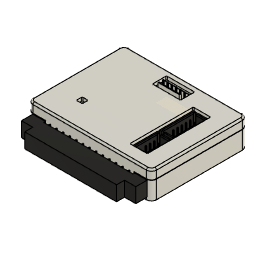
VIC20_Diag_UP_PCB_v0 v8 (Autodesk Fusion 360 design; units mm, degrees)
Autodesk Fusion 360 part; units mm, degrees
(part 1 of 2)
sketch "DXF import" plane through (0, 0, 0) normal (0, 0, 1) x (1, 0, 0) in component "PCB"
  arc A0 (0, 1) -> (1, 0) centre (1, 1) ccw
  line L0 (53, 1) -> (53, 54)
  line L1 (0, 1) -> (0, 54)
  arc A1 (53, 54) -> (52, 55) centre (52, 54) ccw
  line L2 (52, 55) -> (1, 55)
  line L3 (1, 0) -> (52, 0)
  arc A2 (1, 55) -> (0, 54) centre (1, 54) ccw
  arc A3 (52, 0) -> (53, 1) centre (52, 1) ccw
  circle A4 centre (4, 51) radius 3.1
  line L4 (50.18, 0) -> (50.18, -1)
  circle A5 centre (49, 51) radius 3.1
  line L5 (46.72, -1) -> (46.72, 0)
  circle A6 centre (49, 51) radius 1.5875
  line L6 (46.72, 0) -> (46.22, 0)
  line L7 (49.45, 0.1) -> (49.45, -1)
  line L8 (47.45, 0.1) -> (47.45, -1)
  line L9 (46.22, 0) -> (46.22, -1)
  line L10 (50.68, -1) -> (50.68, 0)
  line L11 (50.68, 0) -> (50.18, 0)
  line L12 (31.61, 0.1) -> (31.61, -1)
  circle A7 centre (4, 51) radius 1.5875
  line L13 (22.96, 0) -> (22.46, 0)
  line L14 (7.85, 0.1) -> (7.85, -1)
  line L15 (42.76, -1) -> (42.76, 0)
  line L16 (43.49, 0.1) -> (43.49, -1)
  line L17 (45.49, 0.1) -> (45.49, -1)
  line L18 (30.88, -1) -> (30.88, 0)
  line L19 (7.12, -1) -> (7.12, 0)
  line L20 (22.46, 0) -> (22.46, -1)
  line L21 (7.12, 0) -> (6.62, 0)
  line L22 (35.57, 0.1) -> (35.57, -1)
  line L23 (6.62, 0) -> (6.62, -1)
  line L24 (14.54, 0) -> (14.54, -1)
  line L25 (37.57, 0.1) -> (37.57, -1)
  line L26 (38.8, -1) -> (38.8, 0)
  line L27 (15.04, 0) -> (14.54, 0)
  line L28 (18.5, 0) -> (18.5, -1)
  line L29 (29.65, 0.1) -> (29.65, -1)
  line L30 (30.88, 0) -> (30.38, 0)
  line L31 (27.65, 0.1) -> (27.65, -1)
  line L32 (26.42, 0) -> (26.42, -1)
  line L33 (38.8, 0) -> (38.3, 0)
  line L34 (34.84, 0) -> (34.34, 0)
  line L35 (39.53, 0.1) -> (39.53, -1)
  line L36 (42.26, 0) -> (42.26, -1)
  line L37 (42.76, 0) -> (42.26, 0)
  line L38 (26.92, -1) -> (26.92, 0)
  line L39 (38.3, 0) -> (38.3, -1)
  line L40 (33.61, 0.1) -> (33.61, -1)
  line L41 (34.34, 0) -> (34.34, -1)
  line L42 (26.92, 0) -> (26.42, 0)
  line L43 (30.38, 0) -> (30.38, -1)
  line L44 (34.84, -1) -> (34.84, 0)
  line L45 (41.53, 0.1) -> (41.53, -1)
  line L46 (21.73, 0.1) -> (21.73, -1)
  line L47 (15.77, 0.1) -> (15.77, -1)
  line L48 (11.08, -1) -> (11.08, 0)
  line L49 (23.69, 0.1) -> (23.69, -1)
  line L50 (19.73, 0.1) -> (19.73, -1)
  line L51 (25.69, 0.1) -> (25.69, -1)
  line L52 (19, -1) -> (19, 0)
  line L53 (11.81, 0.1) -> (11.81, -1)
  line L54 (54.17, -6.8) -> (54.17, -11.6)
  line L55 (11.08, 0) -> (10.58, 0)
  line L56 (22.96, -1) -> (22.96, 0)
  line L57 (55.97, -6.8) -> (54.17, -6.8)
  line L58 (-6.03, -6.8) -> (-7.58, -6.8)
  line L59 (59.37, -6.8) -> (55.97, -6.8)
  line L60 (60.92, -6.8) -> (59.37, -6.8)
  line L61 (19, 0) -> (18.5, 0)
  line L62 (9.85, 0.1) -> (9.85, -1)
  line L63 (53.47, 0) -> (53.47, -1)
  line L64 (3.16, -1) -> (3.16, 0)
  line L65 (17.77, 0.1) -> (17.77, -1)
  line L66 (-2.63, -6.8) -> (-2.63, -5.2)
  line L67 (-4.33, 0) -> (-4.33, -2.8667)
  line L68 (57.67, -3.6853) -> (57.67, -3.548)
  line L69 (55.97, -4.2) -> (55.97, -2.6)
  line L70 (59.37, -1.6) -> (59.37, 0)
  line L71 (60.92, 0) -> (59.37, 0)
  line L72 (59.37, 0) -> (57.67, 0)
  line L73 (-4.33, -3.548) -> (-4.33, -3.6853)
  line L74 (-4.33, -4.3667) -> (-4.33, -7.2333)
  line L75 (55.97, -1.6) -> (55.97, 0)
  line L76 (57.67, 0) -> (55.97, 0)
  line L77 (-0.83, -6.8) -> (-2.63, -6.8)
  line L78 (-2.63, -4.2) -> (-2.63, -2.6)
  line L79 (-4.33, -8.7333) -> (-4.33, -11.6)
  line L80 (-4.33, 0) -> (-6.03, 0)
  line L81 (10.58, 0) -> (10.58, -1)
  line L82 (13.81, 0.1) -> (13.81, -1)
  line L83 (5.89, 0.1) -> (5.89, -1)
  line L84 (-2.63, -1.6) -> (-2.63, 0)
  line L85 (-6.03, -1.6) -> (-6.03, 0)
  line L86 (55.97, 0) -> (53.47, 0)
  line L87 (-7.58, 0) -> (-7.58, -6.8)
  line L88 (3.16, 0) -> (2.66, 0)
  line L89 (3.89, 0.1) -> (3.89, -1)
  line L90 (15.04, -1) -> (15.04, 0)
  line L91 (59.37, -4.2) -> (59.37, -2.6)
  line L92 (-6.03, -6.8) -> (-6.03, -5.2)
  line L93 (2.66, 0) -> (2.66, -1)
  line L94 (51.81, 14.73) -> (52.6038, 14.73)
  line L95 (52.6038, 23.62) -> (52.6038, 17.27)
  line L96 (-0.13, 0) -> (-2.63, 0)
  line L97 (60.92, 0) -> (60.92, -6.8)
  line L98 (46.2537, 8.38) -> (44.825, 8.38)
  line L99 (51.81, 17.27) -> (52.6038, 17.27)
  line L100 (-0.83, -11.6) -> (-0.83, -6.8)
  line L101 (-6.03, 0) -> (-7.58, 0)
  line L102 (57.67, -2.8667) -> (57.67, 0)
  line L103 (51.3338, 17.27) -> (51.81, 17.27)
  line L104 (46.2537, 23.62) -> (52.6038, 23.62)
  line L105 (44.6662, 22.35) -> (44.825, 22.35)
  line L106 (51.3338, 9.65) -> (46.2537, 9.65)
  line L107 (44.825, 22.35) -> (44.825, 22.8263)
  line L108 (57.67, -11.6) -> (57.67, -8.7333)
  line L109 (43.3962, 23.62) -> (44.825, 23.62)
  line L110 (51.81, 14.73) -> (51.81, 9.1737)
  line L111 (46.2537, 22.35) -> (46.2537, 22.8263)
  line L112 (57.67, -7.2333) -> (57.67, -4.3667)
  line L113 (44.825, 8.38) -> (43.3962, 8.38)
  line L114 (51.3338, 22.35) -> (51.3338, 17.27)
  line L115 (44.825, 9.65) -> (44.825, 9.1737)
  line L116 (55.97, -6.8) -> (55.97, -5.2)
  line L117 (51.3338, 22.35) -> (51.81, 22.8263)
  line L118 (51.3338, 14.73) -> (51.3338, 9.65)
  line L119 (-4.33, -7.9147) -> (-4.33, -8.052)
  line L120 (53.47, -1) -> (-0.13, -1)
  line L121 (-2.63, -6.8) -> (-6.03, -6.8)
  line L122 (44.6662, 9.65) -> (44.6662, 22.35)
  line L123 (46.2537, 22.35) -> (51.3338, 22.35)
  line L124 (54.17, -11.6) -> (-0.83, -11.6)
  line L125 (57.67, -8.052) -> (57.67, -7.9147)
  line L126 (52.6038, 14.73) -> (52.6038, 8.38)
  line L127 (51.3338, 17.27) -> (51.3338, 14.73)
  line L128 (43.3962, 8.38) -> (43.3962, 23.62)
  line L129 (46.2537, 9.65) -> (44.825, 9.65)
  line L130 (51.3338, 14.73) -> (51.81, 14.73)
  line L131 (-6.03, -4.2) -> (-6.03, -2.6)
  line L132 (52.6038, 17.27) -> (52.6038, 14.73)
  line L133 (52.6038, 8.38) -> (46.2537, 8.38)
  line L134 (44.825, 9.65) -> (44.6662, 9.65)
  line L135 (59.37, -6.8) -> (59.37, -5.2)
  line L136 (44.825, 23.62) -> (46.2537, 23.62)
  line L137 (44.825, 22.35) -> (46.2537, 22.35)
  line L138 (-2.63, 0) -> (-4.33, 0)
  line L139 (-0.13, -1) -> (-0.13, 0)
  arc A8 (43.3962, 35.4763) -> (43.3962, 34.3651) centre (43.3962, 34.9207) ccw
  line L140 (46.2537, 9.1737) -> (51.81, 9.1737)
  line L141 (44.19, 9.1737) -> (44.6662, 9.65)
  arc A9 (43.3962, 10.92) -> (43.3962, 9.65) centre (43.3962, 10.285) ccw
  line L142 (44.825, 22.8263) -> (44.19, 22.8263)
  arc A10 (43.3962, 27.38) -> (43.3962, 26.11) centre (43.3962, 26.745) ccw
  line L143 (44.825, 24.84) -> (43.3962, 24.84)
  line L144 (44.825, 25.6337) -> (44.825, 24.84)
  line L145 (51.81, 25.6337) -> (51.3338, 26.11)
  arc A11 (43.3962, 22.35) -> (43.3962, 21.08) centre (43.3962, 21.715) ccw
  line L146 (44.19, 25.6337) -> (44.825, 25.6337)
  line L147 (44.6662, 26.11) -> (44.6662, 43.89)
  line L148 (44.825, 26.11) -> (44.6662, 26.11)
  line L149 (43.3962, 45.16) -> (44.825, 45.16)
  line L150 (46.2537, 44.3663) -> (46.2537, 45.16)
  line L151 (44.825, 43.89) -> (44.825, 44.3663)
  line L152 (51.81, 9.1737) -> (51.3338, 9.65)
  arc A12 (43.3962, 16.4763) -> (43.3962, 15.3651) centre (43.3962, 15.9207) ccw
  line L153 (46.2537, 22.8263) -> (46.2537, 23.62)
  line L154 (44.19, 9.1737) -> (44.825, 9.1737)
  line L155 (44.825, 9.1737) -> (44.825, 8.38)
  line L156 (51.81, 17.27) -> (51.81, 22.8263)
  line L157 (46.2537, 9.65) -> (46.2537, 9.1737)
  line L158 (46.2537, 22.8263) -> (51.81, 22.8263)
  line L159 (44.6662, 22.35) -> (44.19, 22.8263)
  line L160 (51.3338, 37.0638) -> (51.3338, 32.9362)
  line L161 (51.3338, 37.0638) -> (51.81, 37.0638)
  line L162 (44.825, 44.3663) -> (44.19, 44.3663)
  line L163 (51.3338, 43.89) -> (51.81, 44.3663)
  line L164 (44.825, 43.89) -> (46.2537, 43.89)
  line L165 (46.2537, 25.6337) -> (46.2537, 24.84)
  line L166 (51.3338, 43.89) -> (51.3338, 37.0638)
  line L167 (46.2537, 43.89) -> (46.2537, 44.3663)
  line L168 (51.81, 32.9362) -> (52.6038, 32.9362)
  line L169 (51.3338, 26.11) -> (46.2537, 26.11)
  line L170 (46.2537, 9.1737) -> (46.2537, 8.38)
  line L171 (44.19, 25.6337) -> (44.19, 44.3663)
  line L172 (44.19, 9.1737) -> (44.19, 22.8263)
  line L173 (46.2537, 25.6337) -> (51.81, 25.6337)
  line L174 (44.19, 25.6337) -> (44.6662, 26.11)
  line L175 (44.825, 22.8263) -> (44.825, 23.62)
  line L176 (51.81, 32.9362) -> (51.81, 25.6337)
  line L177 (44.6662, 43.89) -> (44.825, 43.89)
  arc A13 (43.3962, 43.89) -> (43.3962, 42.62) centre (43.3962, 43.255) ccw
  line L178 (44.825, 26.11) -> (44.825, 25.6337)
  line L179 (52.6038, 37.0638) -> (52.6038, 32.9362)
  line L180 (43.3962, 24.84) -> (43.3962, 45.16)
  line L181 (46.2537, 26.11) -> (44.825, 26.11)
  line L182 (44.825, 44.3663) -> (44.825, 45.16)
  line L183 (51.3338, 32.9362) -> (51.3338, 26.11)
  line L184 (51.81, 37.0638) -> (51.81, 44.3663)
  line L185 (46.2537, 45.16) -> (52.6038, 45.16)
  line L186 (46.2537, 43.89) -> (51.3338, 43.89)
  line L187 (52.6038, 32.9362) -> (52.6038, 24.84)
  line L188 (52.6038, 45.16) -> (52.6038, 37.0638)
  line L189 (51.3338, 32.9362) -> (51.81, 32.9362)
  line L190 (44.6662, 43.89) -> (44.19, 44.3663)
  line L191 (52.6038, 24.84) -> (46.2537, 24.84)
  line L192 (46.2537, 44.3663) -> (51.81, 44.3663)
  line L193 (44.825, 45.16) -> (46.2537, 45.16)
  line L194 (46.2537, 24.84) -> (44.825, 24.84)
  line L195 (46.2537, 26.11) -> (46.2537, 25.6337)
  line L196 (51.81, 37.0638) -> (52.6038, 37.0638)
  line L197 (52, 0) -> (59.45, 0)
  line L198 (49.016, 32.206) -> (49.524, 32.206)
  line L199 (45.49, 0.1) -> (45.49, 4)
  line L200 (49.45, 0.1) -> (49.45, 4)
  line L201 (47.95, 3) -> (47.95, 2)
  line L202 (35.57, 0.1) -> (35.57, 4)
  line L203 (48.95, 3) -> (48.95, 2)
  arc A14 (49.45, 4) -> (47.45, 4) centre (48.45, 4) ccw
  line L204 (47.45, 0.1) -> (47.45, 4)
  arc A15 (48.95, 3) -> (47.95, 3) centre (48.45, 3) ccw
  arc A16 (47.95, 2) -> (48.95, 2) centre (48.45, 2) ccw
  arc A17 (29.15, 3) -> (28.15, 3) centre (28.65, 3) ccw
  arc A18 (25.69, 4) -> (23.69, 4) centre (24.69, 4) ccw
  line L205 (37.07, 3) -> (37.07, 2)
  arc A19 (43.99, 2) -> (44.99, 2) centre (44.49, 2) ccw
  line L206 (43.99, 3) -> (43.99, 2)
  line L207 (32.11, 3) -> (32.11, 2)
  arc A20 (44.99, 3) -> (43.99, 3) centre (44.49, 3) ccw
  line L208 (43.49, 0.1) -> (43.49, 4)
  arc A21 (37.07, 3) -> (36.07, 3) centre (36.57, 3) ccw
  arc A22 (40.03, 2) -> (41.03, 2) centre (40.53, 2) ccw
  arc A23 (33.61, 4) -> (31.61, 4) centre (32.61, 4) ccw
  line L209 (40.03, 3) -> (40.03, 2)
  line L210 (25.69, 0.1) -> (25.69, 4)
  arc A24 (28.15, 2) -> (29.15, 2) centre (28.65, 2) ccw
  line L211 (31.61, 0.1) -> (31.61, 4)
  arc A25 (45.49, 4) -> (43.49, 4) centre (44.49, 4) ccw
  line L212 (29.15, 3) -> (29.15, 2)
  arc A26 (25.19, 3) -> (24.19, 3) centre (24.69, 3) ccw
  line L213 (44.99, 3) -> (44.99, 2)
  arc A27 (41.03, 3) -> (40.03, 3) centre (40.53, 3) ccw
  arc A28 (41.53, 4) -> (39.53, 4) centre (40.53, 4) ccw
  line L214 (23.69, 0.1) -> (23.69, 4)
  line L215 (36.07, 3) -> (36.07, 2)
  line L216 (37.57, 0.1) -> (37.57, 4)
  line L217 (41.03, 3) -> (41.03, 2)
  line L218 (27.65, 0.1) -> (27.65, 4)
  line L219 (25.19, 3) -> (25.19, 2)
  line L220 (28.15, 3) -> (28.15, 2)
  line L221 (29.65, 0.1) -> (29.65, 4)
  line L222 (33.61, 0.1) -> (33.61, 4)
  arc A29 (13.81, 4) -> (11.81, 4) centre (12.81, 4) ccw
  line L223 (5.89, 0.1) -> (5.89, 4)
  line L224 (21.23, 3) -> (21.23, 2)
  line L225 (8.35, 3) -> (8.35, 2)
  line L226 (21.73, 0.1) -> (21.73, 4)
  line L227 (9.85, 0.1) -> (9.85, 4)
  line L228 (13.81, 0.1) -> (13.81, 4)
  line L229 (13.31, 3) -> (13.31, 2)
  arc A30 (12.31, 2) -> (13.31, 2) centre (12.81, 2) ccw
  line L230 (3.89, 0.1) -> (3.89, 4)
  line L231 (4.39, 3) -> (4.39, 2)
  arc A31 (29.65, 4) -> (27.65, 4) centre (28.65, 4) ccw
  arc A32 (37.57, 4) -> (35.57, 4) centre (36.57, 4) ccw
  line L232 (19.73, 0.1) -> (19.73, 4)
  arc A33 (9.35, 3) -> (8.35, 3) centre (8.85, 3) ccw
  line L233 (41.53, 0.1) -> (41.53, 4)
  line L234 (11.81, 0.1) -> (11.81, 4)
  arc A34 (36.07, 2) -> (37.07, 2) centre (36.57, 2) ccw
  arc A35 (17.27, 3) -> (16.27, 3) centre (16.77, 3) ccw
  line L235 (33.11, 3) -> (33.11, 2)
  line L236 (15.77, 0.1) -> (15.77, 4)
  line L237 (20.23, 3) -> (20.23, 2)
  line L238 (17.27, 3) -> (17.27, 2)
  line L239 (9.35, 3) -> (9.35, 2)
  arc A36 (13.31, 3) -> (12.31, 3) centre (12.81, 3) ccw
  line L240 (17.77, 0.1) -> (17.77, 4)
  arc A37 (5.39, 3) -> (4.39, 3) centre (4.89, 3) ccw
  line L241 (12.31, 3) -> (12.31, 2)
  arc A38 (8.35, 2) -> (9.35, 2) centre (8.85, 2) ccw
  line L242 (5.39, 3) -> (5.39, 2)
  arc A39 (32.11, 2) -> (33.11, 2) centre (32.61, 2) ccw
  arc A40 (33.11, 3) -> (32.11, 3) centre (32.61, 3) ccw
  line L243 (39.53, 0.1) -> (39.53, 4)
  arc A41 (24.19, 2) -> (25.19, 2) centre (24.69, 2) ccw
  arc A42 (9.85, 4) -> (7.85, 4) centre (8.85, 4) ccw
  arc A43 (21.23, 3) -> (20.23, 3) centre (20.73, 3) ccw
  line L244 (49.524, 16.254) -> (49.016, 16.254)
  line L245 (46.984, 16.254) -> (46.476, 16.254)
  line L246 (49.016, 15.746) -> (49.524, 15.746)
  arc A44 (5.89, 4) -> (3.89, 4) centre (4.89, 4) ccw
  line L247 (46.984, 18.794) -> (46.476, 18.794)
  arc A45 (4.39, 2) -> (5.39, 2) centre (4.89, 2) ccw
  line L248 (46.476, 16.254) -> (46.476, 15.746)
  line L249 (49.016, 13.714) -> (49.016, 13.206)
  line L250 (7.85, 0.1) -> (7.85, 4)
  line L251 (49.524, 15.746) -> (49.524, 16.254)
  line L252 (49.524, 13.714) -> (49.016, 13.714)
  line L253 (16.27, 3) -> (16.27, 2)
  line L254 (46.984, 13.206) -> (46.984, 13.714)
  line L255 (24.19, 3) -> (24.19, 2)
  arc A46 (21.73, 4) -> (19.73, 4) centre (20.73, 4) ccw
  line L256 (46.476, 13.206) -> (46.984, 13.206)
  arc A47 (16.27, 2) -> (17.27, 2) centre (16.77, 2) ccw
  line L257 (46.476, 18.794) -> (46.476, 18.286)
  arc A48 (17.77, 4) -> (15.77, 4) centre (16.77, 4) ccw
  line L258 (46.984, 18.286) -> (46.984, 18.794)
  line L259 (46.476, 15.746) -> (46.984, 15.746)
  arc A49 (20.23, 2) -> (21.23, 2) centre (20.73, 2) ccw
  line L260 (46.984, 15.746) -> (46.984, 16.254)
  line L261 (49.016, 39.826) -> (49.524, 39.826)
  line L262 (49.524, 32.714) -> (49.016, 32.714)
  line L263 (46.984, 35.254) -> (46.476, 35.254)
  line L264 (49.524, 40.334) -> (49.016, 40.334)
  line L265 (46.476, 32.714) -> (46.476, 32.206)
  line L266 (46.476, 35.254) -> (46.476, 34.746)
  line L267 (49.016, 30.174) -> (49.016, 29.666)
  line L268 (49.016, 37.286) -> (49.524, 37.286)
  line L269 (46.476, 18.286) -> (46.984, 18.286)
  line L270 (49.016, 32.714) -> (49.016, 32.206)
  line L271 (46.476, 34.746) -> (46.984, 34.746)
  line L272 (46.476, 32.206) -> (46.984, 32.206)
  line L273 (49.524, 37.286) -> (49.524, 37.794)
  line L274 (46.984, 13.714) -> (46.476, 13.714)
  line L275 (49.016, 13.206) -> (49.524, 13.206)
  line L276 (46.476, 29.666) -> (46.984, 29.666)
  line L277 (49.016, 37.794) -> (49.016, 37.286)
  line L278 (49.524, 30.174) -> (49.016, 30.174)
  line L279 (49.016, 29.666) -> (49.524, 29.666)
  line L280 (49.524, 32.206) -> (49.524, 32.714)
  line L281 (46.476, 30.174) -> (46.476, 29.666)
  line L282 (46.984, 34.746) -> (46.984, 35.254)
  line L283 (46.476, 40.334) -> (46.476, 39.826)
  line L284 (46.476, 37.286) -> (46.984, 37.286)
  line L285 (49.016, 34.746) -> (49.524, 34.746)
  line L286 (46.476, 37.794) -> (46.476, 37.286)
  line L287 (46.984, 39.826) -> (46.984, 40.334)
  line L288 (46.984, 37.794) -> (46.476, 37.794)
  line L289 (49.524, 18.286) -> (49.524, 18.794)
  line L290 (49.524, 13.206) -> (49.524, 13.714)
  line L291 (49.016, 18.286) -> (49.524, 18.286)
  line L292 (49.524, 18.794) -> (49.016, 18.794)
  line L293 (49.016, 35.254) -> (49.016, 34.746)
  line L294 (46.476, 39.826) -> (46.984, 39.826)
  line L295 (46.984, 32.714) -> (46.476, 32.714)
  line L296 (49.524, 37.794) -> (49.016, 37.794)
  line L297 (46.476, 13.714) -> (46.476, 13.206)
  line L298 (49.524, 39.826) -> (49.524, 40.334)
  line L299 (46.984, 37.286) -> (46.984, 37.794)
  line L300 (49.524, 29.666) -> (49.524, 30.174)
  line L301 (49.016, 18.794) -> (49.016, 18.286)
  line L302 (49.016, 40.334) -> (49.016, 39.826)
  line L303 (46.984, 29.666) -> (46.984, 30.174)
  line L304 (46.984, 40.334) -> (46.476, 40.334)
  line L305 (49.016, 16.254) -> (49.016, 15.746)
  line L306 (46.984, 30.174) -> (46.476, 30.174)
  line L307 (49.524, 35.254) -> (49.016, 35.254)
  line L308 (49.524, 34.746) -> (49.524, 35.254)
  line L309 (46.984, 32.206) -> (46.984, 32.714)
sketch "DXF VC20_UP" plane through (0, 0, 0) normal (0, 0, 1) x (1, 0, 0) in component "PCB"
  line L0 (0, 54.9746) -> (0, 0)
  line L1 (53, 55) -> (0.0254, 55)
  arc A0 (0.0254, 55) -> (0, 54.9746) centre (0.0254, 54.9746) ccw
  line L2 (53, 0) -> (53, 55)
  circle A1 centre (49, 51) radius 1.7463
  circle A2 centre (4, 51) radius 3.1789
  circle A3 centre (49, 51) radius 3.1789
  circle A4 centre (4, 51) radius 1.7463
  line L3 (27.841, 46.1455) -> (28.1006, 46.1455)
  arc A5 (27.841, 46.1454) -> (27.5814, 45.8858) centre (27.841, 45.8858) ccw
  line L4 (27.5813, 45.2367) -> (27.5813, 45.8858)
  line L5 (26.6344, 45.6262) -> (27.0239, 45.6262)
  line L6 (25.8744, 44.9771) -> (26.134, 44.9771)
  line L7 (26.6344, 46.1455) -> (27.1537, 46.1455)
  line L8 (27.1537, 44.9771) -> (26.6344, 44.9771)
  arc A6 (27.5814, 45.2367) -> (27.841, 44.9771) centre (27.841, 45.2367) ccw
  line L9 (26.6344, 44.9771) -> (26.6344, 46.1455)
  line L10 (26.0042, 46.1455) -> (26.0042, 44.9771)
  line L11 (25.8744, 46.1455) -> (26.134, 46.1455)
  line L12 (28.1006, 44.9771) -> (27.841, 44.9771)
  line L13 (46.2537, 9.1737) -> (51.81, 9.1737)
  arc A7 (43.3962, 16.4763) -> (43.3962, 15.3651) centre (43.3962, 15.9207) ccw
  line L14 (44.825, 23.62) -> (46.2537, 23.62)
  line L15 (46.2537, 22.35) -> (51.3338, 22.35)
  line L16 (44.825, 43.89) -> (44.825, 44.3663)
  line L17 (46.2537, 22.8263) -> (51.81, 22.8263)
  line L18 (52.6038, 32.9362) -> (52.6038, 24.84)
  line L19 (43.3962, 24.84) -> (43.3962, 45.16)
  line L20 (51.3338, 37.0638) -> (51.81, 37.0638)
  line L21 (52.6038, 24.84) -> (46.2537, 24.84)
  line L22 (44.825, 26.11) -> (44.825, 25.6337)
  line L23 (43.3962, 45.16) -> (44.825, 45.16)
  line L24 (44.825, 45.16) -> (46.2537, 45.16)
  line L25 (52.6038, 37.0638) -> (52.6038, 32.9362)
  line L26 (44.825, 43.89) -> (46.2537, 43.89)
  line L27 (51.81, 37.0638) -> (52.6038, 37.0638)
  line L28 (50.8575, 13.46) -> (51.0162, 13.3012)
  line L29 (46.2537, 26.11) -> (46.2537, 25.6337)
  line L30 (44.825, 24.84) -> (43.3962, 24.84)
  line L31 (46.2537, 43.89) -> (51.3338, 43.89)
  arc A8 (43.3962, 10.92) -> (43.3962, 9.65) centre (43.3962, 10.285) ccw
  line L32 (51.3338, 32.9362) -> (51.3338, 26.11)
  line L33 (44.6662, 26.11) -> (44.6662, 43.89)
  line L34 (51.3338, 26.11) -> (46.2537, 26.11)
  line L35 (51.0162, 13.1425) -> (51.0162, 13.3012)
  line L36 (46.2537, 45.16) -> (52.6038, 45.16)
  line L37 (51.3338, 43.89) -> (51.3338, 37.0638)
  line L38 (51.3338, 37.0638) -> (51.3338, 32.9362)
  line L39 (44.825, 25.6337) -> (44.825, 24.84)
  line L40 (44.19, 9.1737) -> (44.6662, 9.65)
  line L41 (44.19, 9.1737) -> (44.19, 22.8263)
  line L42 (44.825, 44.3663) -> (44.825, 45.16)
  line L43 (46.2537, 24.84) -> (44.825, 24.84)
  line L44 (46.2537, 26.11) -> (44.825, 26.11)
  line L45 (43.3962, 8.38) -> (43.3962, 23.62)
  line L46 (44.825, 26.11) -> (44.6662, 26.11)
  line L47 (51.3338, 32.9362) -> (51.81, 32.9362)
  line L48 (51.0162, 13.3012) -> (51.0162, 13.6187)
  line L49 (51.0162, 13.6187) -> (50.8575, 13.46)
  line L50 (51.81, 32.9362) -> (52.6038, 32.9362)
  line L51 (52.6038, 45.16) -> (52.6038, 37.0638)
  line L52 (44.6662, 43.89) -> (44.825, 43.89)
  line L53 (52.6038, 8.38) -> (46.2537, 8.38)
  line L54 (44.6662, 9.65) -> (44.6662, 22.35)
  line L55 (46.2537, 44.3663) -> (51.81, 44.3663)
  line L56 (51.0162, 29.4437) -> (51.0162, 29.6025)
  line L57 (51.81, 37.0638) -> (51.81, 44.3663)
  line L58 (51.0162, 30.2375) -> (51.0162, 30.3962)
  line L59 (44.19, 25.6337) -> (44.6662, 26.11)
  line L60 (44.6662, 43.89) -> (44.19, 44.3663)
  line L61 (6.635, 17.27) -> (7.27, 16.635)
  line L62 (51.0162, 29.6025) -> (51.0162, 29.7612)
  line L63 (46.2537, 25.6337) -> (51.81, 25.6337)
  line L64 (51.0162, 30.3962) -> (51.0162, 30.555)
  line L65 (46.2537, 25.6337) -> (46.2537, 24.84)
  line L66 (44.19, 25.6337) -> (44.19, 44.3663)
  line L67 (51.0162, 30.2375) -> (50.6987, 29.92)
  line L68 (46.2537, 44.3663) -> (46.2537, 45.16)
  line L69 (5.365, 17.27) -> (4.73, 16.635)
  line L70 (46.2537, 43.89) -> (46.2537, 44.3663)
  line L71 (7.27, 15.365) -> (6.635, 14.73)
  line L72 (50.6987, 29.92) -> (51.0162, 29.6025)
  arc A9 (43.3962, 27.38) -> (43.3962, 26.11) centre (43.3962, 26.745) ccw
  line L73 (51.81, 32.9362) -> (51.81, 25.6337)
  line L74 (50.3812, 29.92) -> (51.0162, 29.285)
  line L75 (51.0162, 29.285) -> (51.0162, 29.4437)
  line L76 (50.8575, 29.92) -> (51.0162, 29.7612)
  line L77 (5.365, 17.27) -> (6.635, 17.27)
  line L78 (51.0162, 30.0787) -> (50.8575, 29.92)
  arc A10 (43.3962, 43.89) -> (43.3962, 42.62) centre (43.3962, 43.255) ccw
  line L79 (44.19, 25.6337) -> (44.825, 25.6337)
  arc A11 (43.3962, 35.4763) -> (43.3962, 34.3651) centre (43.3962, 34.9207) ccw
  line L80 (44.825, 44.3663) -> (44.19, 44.3663)
  line L81 (4.73, 15.365) -> (5.365, 14.73)
  line L82 (51.0162, 30.555) -> (50.3812, 29.92)
  line L83 (51.0162, 29.7612) -> (51.0162, 30.0787)
  line L84 (50.54, 29.92) -> (51.0162, 29.4437)
  line L85 (51.3338, 43.89) -> (51.81, 44.3663)
  line L86 (51.0162, 30.3962) -> (50.54, 29.92)
  line L87 (51.81, 25.6337) -> (51.3338, 26.11)
  line L88 (51.0162, 30.0787) -> (51.0162, 30.2375)
  line L89 (6.635, 14.73) -> (5.365, 14.73)
  line L90 (4.73, 16.635) -> (4.73, 15.365)
  line L91 (7.27, 16.635) -> (7.27, 15.365)
  line L92 (19.38, 46.825) -> (19.38, 53.175)
  line L93 (34.62, 46.825) -> (19.38, 46.825)
  line L94 (33.35, 46.825) -> (33.35, 47.46)
  line L95 (33.35, 47.46) -> (33.35, 48.095)
  line L96 (33.35, 49.0475) -> (33.6675, 48.4125)
  line L97 (33.0325, 48.4125) -> (33.35, 49.0475)
  line L98 (34.62, 53.175) -> (19.38, 53.175)
  line L99 (20.65, 47.46) -> (20.65, 48.095)
  line L100 (20.65, 46.825) -> (20.65, 47.46)
  line L101 (44.825, 22.35) -> (46.2537, 22.35)
  line L102 (33.35, 48.095) -> (20.65, 48.095)
  line L103 (44.825, 22.35) -> (44.825, 22.8263)
  line L104 (44.6662, 22.35) -> (44.825, 22.35)
  line L105 (51.3338, 22.35) -> (51.81, 22.8263)
  line L106 (33.6675, 48.4125) -> (33.0325, 48.4125)
  line L107 (51.0162, 12.825) -> (51.0162, 12.9837)
  line L108 (34.62, 46.825) -> (34.62, 53.175)
  line L109 (51.81, 17.27) -> (52.6038, 17.27)
  line L110 (51.3338, 17.27) -> (51.3338, 14.73)
  line L111 (51.0162, 13.7775) -> (51.0162, 13.9362)
  line L112 (51.0162, 13.9362) -> (51.0162, 14.095)
  line L113 (33.35, 47.46) -> (20.65, 47.46)
  line L114 (51.81, 9.1737) -> (51.3338, 9.65)
  line L115 (51.0162, 12.9837) -> (51.0162, 13.1425)
  line L116 (46.2537, 22.8263) -> (46.2537, 23.62)
  line L117 (44.825, 8.38) -> (43.3962, 8.38)
  line L118 (44.825, 22.8263) -> (44.19, 22.8263)
  line L119 (50.3812, 13.46) -> (51.0162, 12.825)
  line L120 (52.6038, 14.73) -> (52.6038, 8.38)
  line L121 (51.3338, 14.73) -> (51.3338, 9.65)
  line L122 (44.825, 9.1737) -> (44.825, 8.38)
  line L123 (51.0162, 13.9362) -> (50.54, 13.46)
  line L124 (44.6662, 22.35) -> (44.19, 22.8263)
  line L125 (51.0162, 13.6187) -> (51.0162, 13.7775)
  line L126 (46.2537, 8.38) -> (44.825, 8.38)
  line L127 (44.825, 9.65) -> (44.825, 9.1737)
  line L128 (46.2537, 23.62) -> (52.6038, 23.62)
  line L129 (51.81, 14.73) -> (51.81, 9.1737)
  line L130 (52.6038, 17.27) -> (52.6038, 14.73)
  arc A12 (43.3962, 22.35) -> (43.3962, 21.08) centre (43.3962, 21.715) ccw
  line L131 (52.6038, 23.62) -> (52.6038, 17.27)
  line L132 (46.2537, 22.35) -> (46.2537, 22.8263)
  line L133 (43.3962, 23.62) -> (44.825, 23.62)
  line L134 (50.54, 13.46) -> (51.0162, 12.9837)
  line L135 (51.0162, 13.7775) -> (50.6987, 13.46)
  line L136 (50.6987, 13.46) -> (51.0162, 13.1425)
  line L137 (51.0162, 14.095) -> (50.3812, 13.46)
  line L138 (51.3338, 22.35) -> (51.3338, 17.27)
  line L139 (51.3338, 14.73) -> (51.81, 14.73)
  line L140 (46.2537, 9.65) -> (46.2537, 9.1737)
  line L141 (46.2537, 9.65) -> (44.825, 9.65)
  line L142 (46.2537, 9.1737) -> (46.2537, 8.38)
  line L143 (51.81, 17.27) -> (51.81, 22.8263)
  line L144 (51.81, 14.73) -> (52.6038, 14.73)
  line L145 (51.3338, 17.27) -> (51.81, 17.27)
  line L146 (44.825, 22.8263) -> (44.825, 23.62)
  line L147 (44.825, 9.65) -> (44.6662, 9.65)
  line L148 (51.3338, 9.65) -> (46.2537, 9.65)
  line L149 (44.19, 9.1737) -> (44.825, 9.1737)
  line L150 (25.476, 49.746) -> (25.984, 49.746)
  line L151 (33.604, 50.254) -> (33.096, 50.254)
  line L152 (22.936, 50.254) -> (22.936, 49.746)
  line L153 (22.936, 49.746) -> (23.444, 49.746)
  line L154 (28.524, 50.254) -> (28.016, 50.254)
  line L155 (28.016, 50.254) -> (28.016, 49.746)
  line L156 (23.444, 50.254) -> (22.936, 50.254)
  line L157 (25.984, 50.254) -> (25.476, 50.254)
  line L158 (25.984, 49.746) -> (25.984, 50.254)
  line L159 (28.016, 49.746) -> (28.524, 49.746)
  line L160 (23.444, 49.746) -> (23.444, 50.254)
  line L161 (28.524, 49.746) -> (28.524, 50.254)
  line L162 (30.556, 50.254) -> (30.556, 49.746)
  line L163 (31.064, 49.746) -> (31.064, 50.254)
  line L164 (33.096, 50.254) -> (33.096, 49.746)
  line L165 (30.556, 49.746) -> (31.064, 49.746)
  line L166 (31.064, 50.254) -> (30.556, 50.254)
  line L167 (46.984, 18.794) -> (46.476, 18.794)
  line L168 (49.524, 18.794) -> (49.016, 18.794)
  line L169 (49.016, 16.254) -> (49.016, 15.746)
  line L170 (20.904, 50.254) -> (20.396, 50.254)
  line L171 (20.396, 50.254) -> (20.396, 49.746)
  line L172 (46.476, 18.286) -> (46.984, 18.286)
  line L173 (46.476, 13.206) -> (46.984, 13.206)
  line L174 (33.604, 49.746) -> (33.604, 50.254)
  line L175 (20.904, 49.746) -> (20.904, 50.254)
  line L176 (20.396, 49.746) -> (20.904, 49.746)
  line L177 (25.476, 50.254) -> (25.476, 49.746)
  line L178 (49.016, 13.714) -> (49.016, 13.206)
  line L179 (46.984, 13.206) -> (46.984, 13.714)
  line L180 (33.096, 49.746) -> (33.604, 49.746)
  line L181 (49.016, 13.206) -> (49.524, 13.206)
  line L182 (49.524, 13.714) -> (49.016, 13.714)
  line L183 (49.524, 16.254) -> (49.016, 16.254)
  line L184 (49.016, 18.794) -> (49.016, 18.286)
  line L185 (49.016, 15.746) -> (49.524, 15.746)
  line L186 (46.984, 13.714) -> (46.476, 13.714)
  line L187 (46.476, 15.746) -> (46.984, 15.746)
  line L188 (46.476, 32.714) -> (46.476, 32.206)
  line L189 (5.746, 15.746) -> (6.254, 15.746)
  line L190 (49.524, 34.746) -> (49.524, 35.254)
  line L191 (49.524, 35.254) -> (49.016, 35.254)
  line L192 (49.016, 35.254) -> (49.016, 34.746)
  line L193 (49.524, 37.794) -> (49.016, 37.794)
  line L194 (49.524, 29.666) -> (49.524, 30.174)
  line L195 (46.476, 34.746) -> (46.984, 34.746)
  line L196 (5.746, 16.254) -> (5.746, 15.746)
  line L197 (46.984, 40.334) -> (46.476, 40.334)
  line L198 (46.476, 37.794) -> (46.476, 37.286)
  line L199 (46.984, 16.254) -> (46.476, 16.254)
  line L200 (46.476, 16.254) -> (46.476, 15.746)
  line L201 (46.476, 29.666) -> (46.984, 29.666)
  line L202 (46.476, 37.286) -> (46.984, 37.286)
  line L203 (6.254, 15.746) -> (6.254, 16.254)
  line L204 (49.016, 18.286) -> (49.524, 18.286)
  line L205 (46.476, 13.714) -> (46.476, 13.206)
  line L206 (46.984, 34.746) -> (46.984, 35.254)
  line L207 (49.016, 32.206) -> (49.524, 32.206)
  line L208 (49.016, 29.666) -> (49.524, 29.666)
  line L209 (46.984, 30.174) -> (46.476, 30.174)
  line L210 (46.984, 18.286) -> (46.984, 18.794)
  line L211 (49.524, 32.714) -> (49.016, 32.714)
  line L212 (46.984, 29.666) -> (46.984, 30.174)
  line L213 (46.984, 15.746) -> (46.984, 16.254)
  line L214 (49.524, 18.286) -> (49.524, 18.794)
  line L215 (49.524, 32.206) -> (49.524, 32.714)
  line L216 (49.524, 15.746) -> (49.524, 16.254)
  line L217 (49.016, 37.794) -> (49.016, 37.286)
  line L218 (49.524, 13.206) -> (49.524, 13.714)
  line L219 (46.476, 30.174) -> (46.476, 29.666)
  line L220 (49.524, 30.174) -> (49.016, 30.174)
  line L221 (46.476, 32.206) -> (46.984, 32.206)
  line L222 (49.016, 37.286) -> (49.524, 37.286)
  line L223 (49.016, 30.174) -> (49.016, 29.666)
  line L224 (46.984, 37.286) -> (46.984, 37.794)
  line L225 (49.016, 34.746) -> (49.524, 34.746)
  line L226 (46.984, 32.714) -> (46.476, 32.714)
  line L227 (46.476, 35.254) -> (46.476, 34.746)
  line L228 (46.476, 18.794) -> (46.476, 18.286)
  line L229 (46.984, 32.206) -> (46.984, 32.714)
  line L230 (49.016, 32.714) -> (49.016, 32.206)
  line L231 (49.016, 40.334) -> (49.016, 39.826)
  line L232 (6.254, 16.254) -> (5.746, 16.254)
  line L233 (46.476, 39.826) -> (46.984, 39.826)
  line L234 (49.016, 39.826) -> (49.524, 39.826)
  line L235 (46.984, 37.794) -> (46.476, 37.794)
  line L236 (49.524, 40.334) -> (49.016, 40.334)
  line L237 (46.984, 35.254) -> (46.476, 35.254)
  line L238 (49.524, 39.826) -> (49.524, 40.334)
  line L239 (49.524, 37.286) -> (49.524, 37.794)
  line L240 (46.984, 39.826) -> (46.984, 40.334)
  line L241 (46.476, 40.334) -> (46.476, 39.826)
  line L242 (0, 0) -> (53, 0)
  point P0 (4, 51)
  point P1 (8.0962, 52.2288)
  point P2 (48, 16)
  point P3 (48, 35)
  point P4 (6, 16)
  point P5 (49, 51)
  point P6 (27, 50)
  constraint perpendicular L2 L242
extrude "Extrude1" add sketch "DXF import" against normal blind 1.6 contours A0 L0 L1 A1 L2 L3 A2 A3 L6 L7 L8 L11 L12 L13 L14 L16 L17 L21 L22 L25 L27 L29 L30 L31 L33 L34 L35 L37 L40 L42 L45 L46 L47 L49 L50 L51 L53 L55 L61 L62 L65 L82 L83 L88 L89 L199 L200 L202 A14 L204 A18 L208 A23 L210 L211 A25 A28 L214 L216 L218 L221 L222 A29 L223 L226 L227 L228 L230 A31 A32 L232 L233 L234 L236 L240 L243 A42 A44 L250 A46 A48 | L3 L83 L89 L223 L230 A44 | L3 L14 L62 L227 A42 L250 | L3 L7 L8 L200 A14 L204 | L3 L53 L82 A29 L228 L234 | L3 L16 L17 L199 L208 A25 | L3 L47 L65 L236 L240 A48 | L3 L35 L45 A28 L233 L243 | L3 L46 L50 L226 L232 A46 | L3 L22 L25 L202 L216 A32 | L3 L49 L51 A18 L210 L214 | L3 L12 L40 A23 L211 L222 | L3 L29 L31 L218 L221 A31 | A4 | A5 | L94 L99 L103 L127 L130 L132 | L94 L110 L126 L133 L140 L170 | L110 L118 L130 L152 | L106 L140 L152 L157 | L105 L106 L114 L118 L122 L123 L127 L129 L134 L137 | L95 L99 L104 L153 L156 L158 | L98 L115 L129 L155 L157 L170 | L103 L114 L117 L156 | L111 L117 L123 L158 | L109 L113 L128 L142 L154 L155 L172 L175 | L107 L111 L136 L137 L153 L175 | L115 L134 L141 L154 | L122 L141 L159 L172 | L105 L107 L142 L159 | L128 A9 | L128 A11 | L128 A12 | A8 L180 | L143 L144 L146 L149 L162 L171 L180 L182 | A13 L180 | A10 L180 | L150 L151 L164 L167 L182 L193 | L144 L165 L178 L181 L194 L195 | L151 L162 L177 L190 | L150 L184 L185 L188 L192 L196 | L146 L148 L174 L178 | L165 L168 L173 L176 L187 L191 | L147 L148 L160 L164 L166 L169 L177 L181 L183 L186 | L147 L171 L174 L190 | L163 L167 L186 L192 | L145 L169 L173 L195 | L161 L163 L166 L184 | L160 L161 L168 L179 L189 L196 | L145 L176 L183 L189 | L198 L262 L270 L280 | L201 L203 A15 A16 | A17 A24 L212 L220 | L205 A21 L215 A34 | A19 L206 A20 L213 | L207 L235 A39 A40 | A22 L209 A27 L217 | A26 L219 A41 L255 | L224 L237 A43 A49 | L225 A33 L239 A38 | L229 A30 A36 L241 | L231 A37 L242 A45 | A35 L238 L253 A47 | L244 L246 L251 L305 | L245 L248 L259 L260 | L247 L257 L258 L269 | L249 L252 L275 L290 | L254 L256 L274 L297 | L261 L264 L298 L302 | L263 L266 L271 L282 | L265 L272 L295 L309 | L267 L278 L279 L300 | L268 L273 L277 L296 | L276 L281 L303 L306 | L283 L287 L294 L304 | L284 L286 L288 L299 | L285 L293 L307 L308 | L289 L291 L292 L301 makes body 1 in component "PCB"
extrude "Extrude2" add sketch "DXF import" along normal blind 2.2 separate body contours L94 L99 L103 L127 L130 L132 | L105 L106 L114 L118 L122 L123 L127 L129 L134 L137 | L98 L115 L129 L155 L157 L170 | L107 L111 L136 L137 L153 L175 | L150 L151 L164 L167 L182 L193 | L144 L165 L178 L181 L194 L195 | L147 L148 L160 L164 L166 L169 L177 L181 L183 L186 | L160 L161 L168 L179 L189 L196 makes body 2 at (48.8678, 10.8353, 0) makes body 3 at (48.8678, 42.7047, 0) in component "PCB"
extrude "Extrude3" add sketch "DXF import" along normal blind 8.8 separate body contours L94 L110 L126 L133 L140 L170 | L110 L118 L130 L152 | L106 L140 L152 L157 | L95 L99 L104 L153 L156 L158 | L103 L114 L117 L156 | L111 L117 L123 L158 | L109 L113 L128 L142 L154 L155 L172 L175 | L115 L134 L141 L154 | L122 L141 L159 L172 | L105 L107 L142 L159 | L143 L144 L146 L149 L162 L171 L180 L182 | L151 L162 L177 L190 | L150 L184 L185 L188 L192 L196 | L146 L148 L174 L178 | L165 L168 L173 L176 L187 L191 | L147 L171 L174 L190 | L163 L167 L186 L192 | L145 L169 L173 L195 | L161 L163 L166 L184 | L145 L176 L183 L189 makes body 4 at (43.3962, 31.6133, 2.9333) makes body 5 at (50.4871, 8.38, 2.9333) makes body 6 at (52.6038, 42.4613, 5.8667) makes body 7 at (48.3704, 23.62, 2.9333) makes body 8 at (43.3962, 18.54, 2.9333) makes body 9 at (52.6038, 30.2375, 2.9333) in component "PCB"
extrude "Extrude4" add sketch "DXF import" along normal blind 8 contours L198 L262 L270 L280 | L244 L246 L251 L305 | L245 L248 L259 L260 | L247 L257 L258 L269 | L249 L252 L275 L290 | L254 L256 L274 L297 | L261 L264 L298 L302 | L263 L266 L271 L282 | L265 L272 L295 L309 | L267 L278 L279 L300 | L268 L273 L277 L296 | L276 L281 L303 L306 | L283 L287 L294 L304 | L284 L286 L288 L299 | L285 L293 L307 L308 | L289 L291 L292 L301 bodies 3 2 1 in component "PCB"
extrude "Extrude5" add sketch "DXF import" against normal blind 0.5 from surface at -1.6 contours L3 L83 L89 L223 L230 A44 | L3 L83 L89 L120 | L3 L14 L62 L227 A42 L250 | L3 L14 L62 L120 | L3 L7 L8 L120 | L3 L7 L8 L200 A14 L204 | L3 L53 L82 A29 L228 L234 | L3 L53 L82 L120 | L3 L16 L17 L120 | L3 L16 L17 L199 L208 A25 | L3 L47 L65 L236 L240 A48 | L3 L47 L65 L120 | L3 L35 L45 L120 | L3 L35 L45 A28 L233 L243 | L3 L46 L50 L226 L232 A46 | L3 L46 L50 L120 | L3 L22 L25 L120 | L3 L22 L25 L202 L216 A32 | L3 L49 L51 A18 L210 L214 | L3 L49 L51 L120 | L3 L12 L40 L120 | L3 L12 L40 A23 L211 L222 | L3 L29 L31 L218 L221 A31 | L3 L29 L31 L120 bodies 9 5 4 3 6 8 7 in component "PCB"
extrude "Extrude6" add sketch "DXF import" against normal blind 8.8 from surface at 4 contours L3 L64 L88 L93 L120 | L54 L57 L58 L59 L60 L63 L71 L72 L76 L77 L80 L86 L87 L96 L97 L100 L101 L120 L121 L124 L138 L139 L197 | L3 L19 L21 L23 L120 | L3 L4 L10 L11 L120 | L3 L48 L55 L81 L120 | L3 L5 L6 L9 L120 | L3 L24 L27 L90 L120 | L3 L15 L36 L37 L120 | L3 L28 L52 L61 L120 | L3 L26 L33 L39 L120 | L3 L13 L20 L56 L120 | L3 L34 L41 L44 L120 | L3 L32 L38 L42 L120 | L3 L18 L30 L43 L120 bodies 9 4 6 5 8 7 3 in component "PCB"
ref_plane "WorkPlane1" through (0, 0, -4.4) normal (0, 0, 1) x (1, 0, 0) in component "VIC20_diag_up_bottom"
sketch "bottom_shell" plane through (0, 0, -4.4) normal (0, 0, 1) x (1, 0, 0) in component "VIC20_diag_up_bottom"
  circle A0 centre (49, 51) radius 1.5875 construction
  line L0 (1, 0) -> (52, 0) construction
  line L1 (0, 1) -> (0, 54) construction
  line L2 (53, 1) -> (53, 54) construction
  circle A1 centre (4, 51) radius 1.5875 construction
  line L3 (52, 55) -> (1, 55) construction
  line L4 (-7.5, 57.5) -> (60.5, 57.5)
  line L5 (63.5, 54.5) -> (63.5, 3)
  line L6 (60.5, 0) -> (-7.5, 0)
  line L7 (-10.5, 3) -> (-10.5, 54.5)
  arc A2 (-7.5, 57.5) -> (-10.5, 54.5) centre (-7.5, 54.5) ccw
  arc A3 (63.5, 54.5) -> (60.5, 57.5) centre (60.5, 54.5) ccw
  arc A4 (60.5, 0) -> (63.5, 3) centre (60.5, 3) ccw
  arc A5 (-10.5, 3) -> (-7.5, 0) centre (-7.5, 3) ccw
  arc A6 (61.5, 54.5) -> (60.5, 55.5) centre (60.5, 54.5) ccw
  line L8 (-7.5, 55.5) -> (60.5, 55.5)
  arc A7 (-7.5, 55.5) -> (-8.5, 54.5) centre (-7.5, 54.5) ccw
  line L9 (-8.5, 3) -> (-8.5, 54.5)
  arc A8 (-8.5, 3) -> (-7.5, 2) centre (-7.5, 3) ccw
  line L10 (60.5, 2) -> (-7.5, 2)
  arc A9 (60.5, 2) -> (61.5, 3) centre (60.5, 3) ccw
  line L11 (61.5, 54.5) -> (61.5, 3)
  arc A10 (62.3, 54.5) -> (60.5, 56.3) centre (60.5, 54.5) ccw
  line L12 (-7.5, 56.3) -> (60.5, 56.3)
  arc A11 (-7.5, 56.3) -> (-9.3, 54.5) centre (-7.5, 54.5) ccw
  line L13 (-9.3, 3) -> (-9.3, 54.5)
  arc A12 (-9.3, 3) -> (-7.5, 1.2) centre (-7.5, 3) ccw
  arc A13 (60.5, 1.2) -> (62.3, 3) centre (60.5, 3) ccw
  line L14 (62.3, 54.5) -> (62.3, 3)
  circle A14 centre (49, 51) radius 1.75
  circle A15 centre (49, 51) radius 3.5
  circle A16 centre (49, 51) radius 4.25
  circle A17 centre (4, 51) radius 1.75
  circle A18 centre (4, 51) radius 3.5
  circle A19 centre (4, 51) radius 4.25
  circle A20 centre (-4.25, 6.25) radius 1.75
  circle A21 centre (-4.25, 6.25) radius 3
  circle A22 centre (-4.25, 6.25) radius 4
  line L15 (-0.3, 2) -> (-0.3, 0)
  line L16 (53.3, 2) -> (53.3, 0)
  circle A23 centre (57.25, 6.25) radius 1.75
  circle A24 centre (57.25, 6.25) radius 3
  circle A25 centre (57.25, 6.25) radius 4
  line L17 (60.5, 1.2) -> (53, 1.2)
  line L18 (0, 1.2) -> (-7.5, 1.2)
  line L19 (26.5, 55) -> (26.5, 2) construction
  line L20 (-5.7027, 21) -> (58.2376, 21) construction
  line L21 (-2, 22) -> (2, 22)
  line L22 (2, 22) -> (2, 20)
  line L23 (2, 20) -> (-2, 20)
  line L24 (-2, 20) -> (-2, 22)
  line L25 (-0.3, 22) -> (-0.3, 20)
  line L26 (51, 22) -> (55, 22)
  line L27 (55, 22) -> (55, 20)
  line L28 (55, 20) -> (51, 20)
  line L29 (51, 20) -> (51, 22)
  line L30 (54, 22) -> (53.3, 22)
  line L31 (53.3, 22) -> (53.3, 20)
  line L32 (53.3, 20) -> (54, 20)
  point P0 (49, 51)
  point P1 (49, 51)
  dimension "d47" = 57.5
  dimension "d48" = 3
  dimension "d49" = 10.5
  dimension "d50" = 74
  dimension "d51" = 2
  dimension "d53" = 3.5
  dimension "d54" = 7
  dimension "d56" = 3.5
  dimension "d57" = 7
  dimension "d58" = 8.5
  dimension "d59" = 4.25
  dimension "d60" = 4.25
  dimension "d61" = 3.5
  dimension "d62" = 6
  dimension "d63" = 8
  dimension "d64" = 0.3
  dimension "d65" = 0.3
  dimension "d66" = 3.5
  dimension "d67" = 4.25
  dimension "d68" = 4.25
  dimension "d69" = 6
  dimension "d70" = 8
  dimension "d71" = 8.5
  dimension "d72" = 1.2
  dimension "d85" = 19
  dimension "d86" = 4
  dimension "d87" = 2
  dimension "d88" = 0.3
  dimension "d89" = 4
  dimension "d90" = 2
  dimension "d91" = 0.3
  constraint horizontal L4
  constraint vertical L5
  constraint horizontal L6
  constraint vertical L7
  constraint collinear L0 L6
  constraint tangent L4 A2
  constraint tangent L7 A2
  constraint tangent L4 A3
  constraint tangent L5 A3
  constraint equal A2 A3
  constraint tangent L5 A4
  constraint tangent L6 A4
  constraint equal A2 A4
  constraint tangent L6 A5
  constraint tangent L7 A5
  constraint equal A2 A5
  constraint coincident P0 A0.centre
  constraint concentric A14 A15
  constraint concentric A15 A16
  constraint concentric A1 A17
  constraint concentric A1 A18
  constraint concentric A17 A19
  constraint concentric A20 A21
  constraint concentric A20 A22
  constraint coincident L10 L15.start
  constraint coincident L6 L15.end
  constraint perpendicular L6 L15
  constraint coincident L10 L16.start
  constraint coincident L6 L16.end
  constraint perpendicular L6 L16
  constraint concentric A23 A24
  constraint concentric A24 A25
  constraint concentric A3 A10
  constraint parallel L4 L12
  constraint concentric A2 A11
  constraint parallel L7 L13
  constraint concentric A5 A12
  constraint parallel L6 L17
  constraint concentric A4 A13
  constraint parallel L5 L14
  constraint tangent A10 L14
  constraint tangent A13 L17
  constraint tangent A10 L12
  constraint tangent A13 L14
  constraint tangent L12 A11
  constraint tangent A11 L13
  constraint tangent A12 L17
  constraint tangent L13 A12
  constraint coincident L2 L17.end
  constraint coincident L1 L18.start
  constraint collinear L17 L18
  constraint midpoint L3 L19.start
  constraint midpoint L10 L19.end
  constraint perpendicular L2 L20
  constraint horizontal L21
  constraint vertical L22
  constraint horizontal L23
  constraint vertical L24
  constraint symmetric L20 L21 L23
  constraint symmetric L1 L22 L24
  constraint coincident L21 L25.start
  constraint coincident L23 L25.end
  constraint perpendicular L23 L25
  constraint horizontal L26
  constraint vertical L27
  constraint horizontal L28
  constraint vertical L29
  constraint horizontal L30
  constraint vertical L31
  constraint horizontal L32
  constraint coincident L28 L31.end
  constraint coincident L26 L30.start
  constraint symmetric L20 L26 L28
  constraint symmetric L2 L27 L29
  measures "d47" distance of L4 L6
  measures "d48" radius of A2
  measures "d49" distance of L1 L7
  measures "d50" distance of L5 L7
  measures "d53" diameter of A14
  measures "d54" diameter of A15
  measures "d56" diameter of A17
  measures "d57" diameter of A18
  measures "d58" diameter of A19
  measures "d59" distance of L1 A20.centre
  measures "d60" distance of L10 A20.centre
  measures "d61" diameter of A20
  measures "d62" diameter of A21
  measures "d63" diameter of A22
  measures "d64" distance of L1 L15
  measures "d65" distance of L2 L16
  measures "d66" diameter of A23
  measures "d67" distance of L2 A23.centre
  measures "d68" distance of L10 A23.centre
  measures "d69" diameter of A24
  measures "d70" diameter of A25
  measures "d71" diameter of A16
  measures "d72" distance of L7 L13
  measures "d85" distance of L10 L20
  measures "d86" distance of L22 L24
  measures "d87" distance of L21 L23
  measures "d88" distance of L1 L25
  measures "d89" distance of L27 L29
  measures "d90" distance of L26 L28
  measures "d91" distance of L2 L31
extrude "Extrude1'" add sketch "bottom_shell" against normal blind 2 separate body contours L4 L5 L6 L7 A2 A3 A4 A5 A10 L12 A11 L13 A12 A13 L14 L15 L16 L17 L18 | L6 L10 L15 L16 | A6 L8 A7 L9 A8 L10 A9 L11 A10 L12 A11 L13 A12 A13 L14 L15 L16 L17 L18 | A6 L8 A7 L9 A8 L10 A9 L11 | A16 | A19 | A22 | A25 | L21 L23 L24 L25 | L21 L22 L23 L25 | L26 L28 L29 L31 | L26 L27 L28 L30 L31 L32 makes body 10 in component "VIC20_diag_up_bottom"
extrude "Extrude2'" add sketch "bottom_shell" along normal blind 1 contours L6 L10 L15 L16 bodies 10 in component "VIC20_diag_up_bottom"
extrude "Extrude3'" add sketch "bottom_shell" along normal blind 9.7 contours A6 L8 A7 L9 A8 L10 A9 L11 A10 L12 A11 L13 A12 A13 L14 L15 L16 L17 L18 bodies 10 in component "VIC20_diag_up_bottom"
extrude "Extrude4'" add sketch "bottom_shell" along normal blind 8.7 contours L4 L5 L6 L7 A2 A3 A4 A5 A10 L12 A11 L13 A12 A13 L14 L15 L16 L17 L18 bodies 10 in component "VIC20_diag_up_bottom"
extrude "Extrude5'" add sketch "bottom_shell" along normal blind 2.8 contours A15 | A16 | A18 | A19 | L21 L22 L23 L25 | L26 L28 L29 L31 bodies 10 in component "VIC20_diag_up_bottom"
extrude "Extrude6'" add sketch "bottom_shell" along normal blind 4.4 contours A21 | A22 | A24 | A25 | L21 L23 L24 L25 | L26 L27 L28 L30 L31 L32 bodies 10 in component "VIC20_diag_up_bottom"
chamfer "Chamfer1" distance 1.3 angle 45 2 edges at (0.0376, 49.4631, -1.6) (45.0376, 49.4631, -1.6) on bodies 10 in component "VIC20_diag_up_bottom"
fillet "Fillet1" radius 0.5 4 edges at (-7.9793, 7.6965, -4.4) (0.0376, 52.5369, -4.4) (45.0376, 52.5369, -4.4) (53.5207, 4.8035, 0) on bodies 10 in component "VIC20_diag_up_bottom"
fillet "Fillet2" radius 0.5 4 edges at (0, 20, -4.4) (2, 21, -4.4) (0, 22, -4.4) (-2, 21, -4.4) on bodies 10 in component "VIC20_diag_up_bottom"
fillet "Fillet3" radius 0.5 4 edges at (51, 21, -4.4) (53, 22, -4.4) (55, 21, -4.4) (53, 20, -4.4) on bodies 10 in component "VIC20_diag_up_bottom"
fillet "Fillet4" radius 0.5 1 edges at (53.5207, 7.6965, -4.4) on bodies 10 in component "VIC20_diag_up_bottom"
fillet "Fillet5" radius 0.5 1 edges at (-7.9793, 4.8035, 0) on bodies 10 in component "VIC20_diag_up_bottom"
ref_plane "WorkPlane1" through (0, 0, 8) normal (0, 0, 1) x (1, 0, 0) in component "VIC20_diag_up_top"